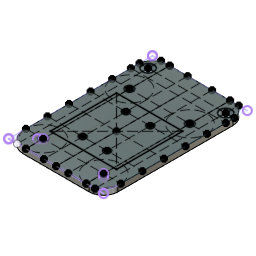
Laser Carriage - Laser Side (Autodesk Fusion 360 design; units mm, degrees)
Autodesk Fusion 360 part; units mm, degrees
sketch "Sketch1" plane through (0, 0, 0) normal (0, 0, 1) x (1, 0, 0) in component "Laser Carriage - Laser Side"
  line L0 (0, 0) -> (66, 0)
  line L1 (66, 0) -> (66, 100)
  line L2 (66, 100) -> (0, 100)
  line L3 (0, 100) -> (0, 0)
  dimension "d1" = 66
  dimension "d2" = 100
  constraint horizontal L0
  constraint vertical L1
  constraint horizontal L2
  constraint vertical L3
  constraint coincident L0.start L3.end
  measures "d1" distance of L0.start L0.end
  measures "d2" distance of L0.start L2.end
extrude "Extrude1" add sketch "Sketch1" along normal blind 4 in component "Laser Carriage - Laser Side"
sketch "Sketch2" plane through (0, 0, 4) normal (0, 0, 1) x (-1, 0, 0) in component "Laser Carriage - Laser Side"
  line L0 (0, -100) -> (0, 0)
  line L1 (0, 0) -> (-66, 0)
  line L2 (-66, 0) -> (-66, -100)
  line L3 (-66, -100) -> (0, -100)
  line L4 (-12, -100) -> (-12, 0) construction
  line L5 (-54, -100) -> (-54, 0) construction
  line L6 (0, -12) -> (-66, -12) construction
  line L7 (0, -72) -> (-66, -72) construction
  circle A0 centre (-12, -72) radius 12 construction
  circle A1 centre (-54, -72) radius 12 construction
  circle A2 centre (-12, -72) radius 2.65
  circle A3 centre (-54, -72) radius 2.65
  line L8 (-12, 0) -> (-12, -100) construction
  line L9 (-54, 0) -> (-54, -100) construction
  circle A4 centre (-12, -12) radius 12 construction
  circle A5 centre (-54, -12) radius 12 construction
  circle A6 centre (-12, -12) radius 2.65
  circle A7 centre (-54, -12) radius 2.65
  line L10 (0, -85) -> (-66, -85) construction
  line L11 (-33, -85) -> (-33, 0) construction
  dimension "d8" = 12
  dimension "d13" = 24
  dimension "d14" = 24
  dimension "d16" = 5.3
  dimension "d17" = 5.3
  dimension "d40" = 60
  dimension "d53" = 24
  dimension "d54" = 24
  dimension "d55" = 5.3
  dimension "d56" = 5.3
  dimension "d234" = 13
  dimension "d237" = 42
  dimension "d238" = 21
  dimension "d239" = 42
  dimension "d240" = 21
  constraint coincident L3 L4.start
  constraint coincident L1 L4.end
  constraint perpendicular L1 L4
  constraint coincident L3 L5.start
  constraint coincident L1 L5.end
  constraint perpendicular L1 L5
  constraint coincident L1 L11.end
  constraint coincident L0 L6.start
  constraint coincident L2 L6.end
  constraint perpendicular L2 L6
  constraint coincident L0 L7.start
  constraint coincident L2 L7.end
  constraint perpendicular L2 L7
  constraint coincident L7 A0.centre
  constraint coincident L4 A0.centre
  constraint coincident L7 A1.centre
  constraint coincident L5 A1.centre
  constraint concentric A0 A2
  constraint concentric A1 A3
  constraint perpendicular L3 L8
  constraint perpendicular L3 L9
  constraint coincident L8 A4.centre
  constraint coincident L6 A4.centre
  constraint coincident L9 A5.centre
  constraint coincident L6 A5.centre
  constraint concentric A4 A6
  constraint concentric A5 A7
  constraint coincident L0 L10.start
  constraint coincident L2 L10.end
  constraint perpendicular L2 L10
  constraint midpoint L10 L11.start
  measures "d8" distance of L1 L6
  measures "d13" diameter of A0
  measures "d14" diameter of A1
  measures "d16" diameter of A2
  measures "d17" diameter of A3
  measures "d40" distance of L6 L7
  measures "d53" diameter of A4
  measures "d54" diameter of A5
  measures "d55" diameter of A6
  measures "d56" diameter of A7
  measures "d234" distance of A0.centre L10
  measures "d237" distance of L4 L5
  measures "d238" distance of L4 L11
  measures "d239" distance of L8 L9
  measures "d240" distance of L8 L11
extrude "Extrude2" cut sketch "Sketch2" against normal up to surface (4 mm away) contours A2 | A3 | A6 | A7 in component "Laser Carriage - Laser Side"
fillet "Fillet5" radius 10 2 edges at (0, 100, 2) (66, 100, 2) in component "Laser Carriage - Laser Side"
fillet "Fillet5" radius 10 2 edges at (66, 0, 2) (0, 0, 2) in component "Laser Carriage - Laser Side"
sketch "Sketch16" plane through (0, 0, 4) normal (0, 0, 1) x (-1, 0, 0) in component "Laser Carriage - Laser Side"
  circle A0 centre (-54, -72) radius 2.65
  circle A1 centre (-12, -72) radius 2.65
  arc A2 (-66, -90) -> (-56, -100) centre (-56, -90) ccw
  line L0 (-56, -100) -> (-10, -100)
  arc A3 (-10, -100) -> (0, -90) centre (-10, -90) ccw
  line L1 (0, -90) -> (0, -10)
  line L2 (-10, 0) -> (-56, 0)
  line L3 (-66, -10) -> (-66, -90)
  line L4 (-33, -100) -> (-33, 0) construction
  line L5 (0, -42) -> (-66, -42) construction
  line L6 (-41.5, -100) -> (-41.5, 0) construction
  line L7 (-24.5, -100) -> (-24.5, 0) construction
  line L8 (0, -57) -> (-66, -57) construction
  line L9 (0, -27) -> (-66, -27) construction
  circle A4 centre (-24.5, -57) radius 2.25
  circle A5 centre (-41.5, -57) radius 2.25
  circle A6 centre (-24.5, -27) radius 2.25
  circle A7 centre (-41.5, -27) radius 2.25
  arc A8 (0, -10) -> (-10, 0) centre (-10, -10) ccw
  arc A9 (-56, 0) -> (-66, -10) centre (-56, -10) ccw
  line L10 (-56, -65) -> (-10, -65)
  line L11 (-10, -65) -> (-10, -19)
  line L12 (-10, -19) -> (-56, -19)
  line L13 (-56, -19) -> (-56, -65)
  line L14 (-56, -65) -> (-10, -19) construction
  line L15 (-10, -65) -> (-56, -19) construction
  circle A10 centre (-12, -12) radius 2.65
  circle A11 centre (-54, -12) radius 2.65
  line L16 (0, -91) -> (-66, -91) construction
  line L17 (-66, -100) -> (0, -100) construction
  line L18 (-6, 0) -> (-6, -100) construction
  line L19 (0, -100) -> (0, 0) construction
  line L20 (-60, 0) -> (-60, -100) construction
  circle A12 centre (-6, -91) radius 4
  circle A13 centre (-60, -91) radius 4
  line L21 (0, 0) -> (-66, 0)
  point P0 (-33, -42)
  dimension "d246" = 15
  dimension "d247" = 15
  dimension "d248" = 8.5
  dimension "d249" = 8.5
  dimension "d250" = 4.5
  dimension "d251" = 4.5
  dimension "d252" = 4.5
  dimension "d253" = 4.5
  dimension "d262" = 46
  dimension "d263" = 46
  dimension "d268" = 6
  dimension "d269" = 6
  dimension "d270" = 8
  dimension "d271" = 8
  dimension "d272" = 42
  dimension "d273" = 91
  constraint midpoint L0 L4.start
  constraint coincident L1 L5.start
  constraint perpendicular L4 L5
  constraint coincident L0 L6.start
  constraint coincident L2 L6.end
  constraint perpendicular L2 L6
  constraint coincident L2 L7.end
  constraint perpendicular L2 L7
  constraint coincident L1 L8.start
  constraint coincident L3 L8.end
  constraint perpendicular L3 L8
  constraint coincident L1 L9.start
  constraint coincident L3 L9.end
  constraint perpendicular L3 L9
  constraint coincident L8 A4.centre
  constraint coincident L7 A4.centre
  constraint coincident L8 A5.centre
  constraint coincident L6 A5.centre
  constraint coincident L7 A6.centre
  constraint coincident L9 A6.centre
  constraint coincident L9 A7.centre
  constraint coincident L6 A7.centre
  constraint coincident L3 L5.end
  constraint horizontal L10
  constraint perpendicular L10 L11
  constraint parallel L10 L12
  constraint parallel L11 L13
  constraint coincident L14 P0
  constraint coincident L15 P0
  constraint midpoint L5 P0
  constraint coincident L0 L7.start
  constraint coincident L1 L16.start
  constraint coincident L3 L16.end
  constraint perpendicular L3 L16
  constraint coincident L17 L18.end
  constraint coincident L2 L20.start
  constraint coincident L17 L20.end
  constraint coincident L16 A12.centre
  constraint coincident L18 A12.centre
  constraint coincident L16 A13.centre
  constraint coincident L20 A13.centre
  measures "d246" distance of L5 L8
  measures "d247" distance of L5 L9
  measures "d248" distance of L4 L7
  measures "d249" distance of L4 L6
  measures "d250" diameter of A4
  measures "d251" diameter of A5
  measures "d252" diameter of A6
  measures "d253" diameter of A7
  measures "d262" distance of L11.end L12.end
  measures "d263" distance of L10.end L11.end
  measures "d268" distance of L18 L19
  measures "d269" distance of L3 L20
  measures "d270" diameter of A12
  measures "d271" diameter of A13
  measures "d272" distance of L5 L21
  measures "d273" distance of L2 L16
extrude "Extrude17" cut sketch "Sketch16" against normal up to surface (4 mm away) contours A4 | A5 | A6 | A7 | A12 | A13 in component "Laser Carriage - Laser Side"
component "Laser Carriage - Laser Side" placed x (1, 0, 0) y (0, 1, 0) z (0, 0, 1) at (0, 0, 0)
named bodies: "Laser Carriage - Laser Side"
